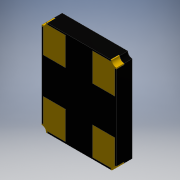
# Autodesk Inventor part: 403C
Saved by Autodesk Inventor 2016 (Build 200138000, 138)
## iProperties
Created: 2016-07-05
Part Number: 403C
Material: Generic
Document SubType Name: Modeling
Designer: Jonathan
Density: 1 g/cm^3
Appearance: Default
Author: Jonathan
Autodesk Inventor part; units mm, degrees
ref_plane "YZ Plane" through (0, 0, 0) normal (1, 0, 0) x (0, 1, 0)
ref_plane "XZ Plane" through (0, 0, 0) normal (0, 1, 0) x (-1, 0, 0)
ref_plane "XY Plane" through (0, 0, 0) normal (0, 0, 1) x (1, 0, 0)
sketch "Sketch1" plane through (0, 0, 0) normal (0, 1, 0) x (-1, 0, 0)
  line L0 (1.1, 1.6) -> (-1.1, 1.6)
  line L1 (-1.25, 1.45) -> (-1.25, -1.45)
  line L2 (-1.1, -1.6) -> (1.1, -1.6)
  line L3 (1.25, -1.45) -> (1.25, 1.45)
  arc A0 (1.25, -1.45) -> (1.1, -1.6) centre (1.25, -1.6) ccw
  arc A1 (1.1, 1.6) -> (1.25, 1.45) centre (1.25, 1.6) ccw
  arc A2 (-1.1, -1.6) -> (-1.25, -1.45) centre (-1.25, -1.6) ccw
  arc A3 (-1.25, 1.45) -> (-1.1, 1.6) centre (-1.25, 1.6) ccw
  point P0 (0, 0)
  point P1 (1.25, 0)
  point P2 (-1.25, 0)
  point P3 (0, 1.6)
  point P4 (0, -1.6)
  dimension "d2" = 3.2
  dimension "d3" = 2.5
  dimension "d4" = 0.15
  constraints: 8 end point, 8 point on circle, 5 horizontal alignment, 5 vertical alignment, 4 centre point, 4 midpoint, 3 equal radius, 2 parallel, 1 horizontal, 1 perpendicular
  measures "d2" distance between parallel lines of L2 L0
  measures "d3" distance between parallel lines of L1 L3
  measures "d4" radius of A0
extrude "Extrusion1" add sketch "Sketch1" along normal blind 0.5333
sketch "Sketch3" plane through (0, 0.5333, 0) normal (0, 1, 0) x (1, 0, 0)
  line L0 (0.95, 1.5) -> (-0.95, 1.5)
  line L1 (-1.15, 1.3) -> (-1.15, -1.3)
  line L2 (-0.95, -1.5) -> (0.95, -1.5)
  line L3 (1.15, -1.3) -> (1.15, 1.3)
  arc A0 (1.15, 1.3) -> (0.95, 1.5) centre (0.95, 1.3) ccw
  arc A1 (-0.95, 1.5) -> (-1.15, 1.3) centre (-0.95, 1.3) ccw
  arc A2 (-1.15, -1.3) -> (-0.95, -1.5) centre (-0.95, -1.3) ccw
  arc A3 (0.95, -1.5) -> (1.15, -1.3) centre (0.95, -1.3) ccw
  point P0 (0, 0)
  point P1 (0, 0)
  point P2 (0, 1.5)
  point P3 (1.15, 0)
  dimension "d12" = 3
  dimension "d13" = 2.3
  dimension "d14" = 0.2
  constraints: 8 end point, 8 point on circle, 8 tangent, 4 centre point, 3 equal radius, 2 horizontal alignment, 2 midpoint, 2 parallel, 2 vertical alignment, 1 horizontal, 1 perpendicular
  measures "d12" distance between parallel lines of L2 L0
  measures "d13" distance between parallel lines of L1 L3
  measures "d14" radius of A0
extrude "Extrusion7" cut sketch "Sketch3" against normal blind 0.001
extrude "Extrusion3" add sketch "Sketch3" against normal blind 0.001 separate body
sketch "Sketch2" plane through (0, 0.5333, 0) normal (0, 1, 0) x (1, 0, 0)
  line L0 (0.85, 1.4) -> (-0.85, 1.4)
  line L1 (-1.05, 1.2) -> (-1.05, -1.2)
  line L2 (-0.85, -1.4) -> (0.85, -1.4)
  line L3 (1.05, -1.2) -> (1.05, 1.2)
  arc A0 (1.05, 1.2) -> (0.85, 1.4) centre (0.85, 1.2) ccw
  arc A1 (-0.85, 1.4) -> (-1.05, 1.2) centre (-0.85, 1.2) ccw
  arc A2 (-1.05, -1.2) -> (-0.85, -1.4) centre (-0.85, -1.2) ccw
  arc A3 (0.85, -1.4) -> (1.05, -1.2) centre (0.85, -1.2) ccw
  point P0 (0, 0)
  point P1 (0, 1.4)
  point P2 (1.05, 0)
  dimension "d7" = 2.8
  dimension "d8" = 2.1
  dimension "d9" = 0.2
  constraints: 8 end point, 8 point on circle, 8 tangent, 4 centre point, 3 equal radius, 2 midpoint, 2 parallel, 1 horizontal, 1 horizontal alignment, 1 perpendicular, 1 vertical alignment
  measures "d7" distance between parallel lines of L2 L0
  measures "d8" distance between parallel lines of L1 L3
  measures "d9" radius of A0
extrude "Extrusion2" add sketch "Sketch2" along normal blind 0.1 bodies 2
sketch "Sketch4" plane through (0, 0.6333, 0) normal (0, 1, 0) x (1, 0, 0)
  line L0 (0.8, 1.35) -> (-0.8, 1.35)
  line L1 (-1, 1.15) -> (-1, -1.15)
  line L2 (-0.8, -1.35) -> (0.8, -1.35)
  line L3 (1, -1.15) -> (1, 1.15)
  arc A0 (1, 1.15) -> (0.8, 1.35) centre (0.8, 1.15) ccw
  arc A1 (-0.8, 1.35) -> (-1, 1.15) centre (-0.8, 1.15) ccw
  arc A2 (-1, -1.15) -> (-0.8, -1.35) centre (-0.8, -1.15) ccw
  arc A3 (0.8, -1.35) -> (1, -1.15) centre (0.8, -1.15) ccw
  point P0 (0, 0)
  point P1 (0, 0)
  point P2 (0, 1.35)
  point P3 (1, 0)
  dimension "d17" = 2.7
  dimension "d18" = 2
  dimension "d19" = 0.2
  constraints: 8 end point, 8 point on circle, 8 tangent, 4 centre point, 3 equal radius, 2 midpoint, 2 parallel, 1 coincident, 1 horizontal, 1 horizontal alignment, 1 perpendicular, 1 vertical alignment
  measures "d17" distance between parallel lines of L2 L0
  measures "d18" distance between parallel lines of L1 L3
  measures "d19" radius of A0
extrude "Extrusion4" add sketch "Sketch4" along normal blind 0.1 separate body
fillet "Fillet1" radius 0.05 8 edges at (-0.9914, 0.5333, -1.3414) (0, 0.5333, -1.4) (0.9914, 0.5333, -1.3414) (1.05, 0.5333, 0) (0.9914, 0.5333, 1.3414) (0, 0.5333, 1.4) (-0.9914, 0.5333, 1.3414) (-1.05, 0.5333, 0)
sketch "Sketch5" plane through (0, 0, 0) normal (0, -1, 0) x (1, 0, 0)
  arc A0 (-1.06, -1.6) -> (-1.25, -1.41) centre (-1.25, -1.6) ccw
  arc A1 (-1.1, -1.6) -> (-1.25, -1.45) centre (-1.25, -1.6) ccw projected
  line L0 (-1.25, -1.45) -> (-1.25, 1.45) projected
  line L1 (1.1, -1.6) -> (-1.1, -1.6) projected
  point P0 (0, 0)
  dimension "d23" = 0.38
  constraints: 2 point on circle, 2 point on line, 1 centre point, 1 concentric
  measures "d23" diameter of A0
extrude "Extrusion10" cut sketch "Sketch5" against normal blind 0.2667 bodies 1
sketch "Sketch6" plane through (0, 0, 0) normal (0, -1, 0) x (1, 0, 0)
  line L0 (-0.45, -0.6) -> (-1.2, -0.6)
  line L1 (-1.2, -0.6) -> (-1.2, -1.4167)
  line L2 (-1.0667, -1.55) -> (-0.45, -1.55)
  line L3 (-0.45, -1.55) -> (-0.45, -0.6)
  line L4 (1.1, -1.6) -> (-1.1, -1.6) projected
  line L5 (-1.25, -1.45) -> (-1.25, 1.45) projected
  arc A0 (-1.06, -1.6) -> (-1.25, -1.41) centre (-1.25, -1.6) ccw projected
  point P0 (0, 0)
  dimension "d26" = 1
  dimension "d27" = 0.8
  dimension "d28" = 0.05
  dimension "d29" = 0.05
  constraints: 8 end point, 2 parallel, 2 point on circle, 1 horizontal, 1 perpendicular
  measures "d26" distance between parallel lines of L4 L0
  measures "d27" distance between parallel lines of L5 L3
  measures "d28" distance between parallel lines of L1 L5
  measures "d29" distance between parallel lines of L4 L2
extrude "Extrusion11" cut sketch "Sketch6" against normal blind 0.04 bodies 1
mirror "Mirror4" about plane through (0, 0, 0) normal (0, 0, 1) of "Extrusion10", "Extrusion11" bodies 1
mirror "Mirror5" about plane through (0, 0, 0) normal (1, 0, 0) of "Extrusion10", "Extrusion11", "Mirror4" bodies 1
extrude "Extrusion12" add sketch "Sketch6" against normal blind 0.04 separate body
extrude "Extrusion13" add sketch "Sketch5" against normal blind 0.2667 bodies 4
mirror "Mirror6" about plane through (0, 0, 0) normal (1, 0, 0) of "Extrusion12", "Extrusion13" bodies 4
mirror "Mirror7" about plane through (0, 0, 0) normal (0, 0, 1) of "Mirror6", "Extrusion13", "Extrusion12" bodies 4
body "Solid1"
body "Solid2"
body "Solid3"
body "Solid5"
